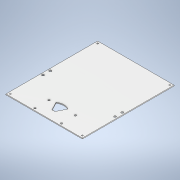
# Autodesk Inventor part: s_carbon_plate1
Saved by Autodesk Inventor 2022 (Build 260153000, 153)
## iProperties
Created: 2021-08-20
Part Number: s_carbon_plate1
Material: ABS プラスチック
Document SubType Name: Sheet Metal
Designer: yuta0
Density: 1.06 g/cm^3
Sheet Metal Rule: Default_mm
Appearance: 滑らか - 白
Author: yuta0
Autodesk Inventor part; units mm, degrees
ref_plane "YZ Plane" through (0, 0, 0) normal (1, 0, 0) x (0, 1, 0)
ref_plane "XZ Plane" through (0, 0, 0) normal (0, 1, 0) x (-1, 0, 0)
ref_plane "XY Plane" through (0, 0, 0) normal (0, 0, 1) x (1, 0, 0)
sketch "スケッチ1" plane through (0, 0, 0) normal (0, 1, 0) x (-1, 0, 0)
  line L0 (-87.5, 105) -> (87.5, 105)
  line L1 (87.5, 105) -> (87.5, -105)
  line L2 (87.5, -105) -> (-87.5, -105)
  line L3 (-87.5, -105) -> (-87.5, 105)
  line L4 (-87.5, 105) -> (87.5, -105) construction
  line L5 (87.5, 105) -> (-87.5, -105) construction
  point P0 (0, 0)
  dimension "d0" = 210
  dimension "d1" = 175
  measures "d0" distance of L0.end L1.end
  measures "d1" distance of L0.start L0.end
extrude "プレート1" add sketch "スケッチ1" along normal blind 2
sketch "スケッチ5" plane through (0, 2, 0) normal (0, 1, 0) x (1, 0, 0)
  line L0 (-26, -100) -> (34.6, -100)
  line L1 (34.6, -100) -> (34.6, -68)
  line L2 (34.6, -68) -> (-26, -68)
  line L3 (-26, -68) -> (-26, -100)
  line L4 (-26, -100) -> (34.6, -68) construction
  line L5 (34.6, -100) -> (-26, -68) construction
  line L6 (87.5, -105) -> (-87.5, -105) projected
  point P0 (0, 0)
  point P1 (0, -84)
  point P2 (4.3, -84)
  point P3 (4.3, -84)
  dimension "d31" = 60.6
  dimension "d32" = 26
  dimension "d33" = 32
  dimension "d34" = 21
  constraints: 12 end point, 3 midpoint, 2 parallel, 1 horizontal, 1 horizontal alignment, 1 perpendicular, 1 vertical alignment
  measures "d31" distance of L1.end L2.end
  measures "d32" distance from line of L3 point (0, -84)
  measures "d33" distance of L0.end L1.end
  measures "d34" distance from line of L6 point (0, -84)
hole "穴3" at (34.6, 2, 68) at (34.6, 2, 100) at (-26, 2, 68) at (-26, 2, 100) direction (0, -1, 0) diameter 4.3 end through all clearance for "Socket Head Cap Screw" size "M4" standard "Ansi Metric M Profile"
sketch "スケッチ6" plane through (0, 2, 0) normal (0, 1, 0) x (1, 0, 0)
  line L0 (-87.5, -251.5284) -> (85.7224, 84.4449)
  line L1 (85.7224, 84.4449) -> (87.5, 83.5284)
  line L2 (87.5, 83.5284) -> (-85.7224, -252.4449)
  line L3 (-85.7224, -252.4449) -> (-87.5, -251.5284)
  line L4 (-87.5, -251.5284) -> (87.5, 83.5284) construction
  line L5 (85.7224, 84.4449) -> (-85.7224, -252.4449) construction
  line L6 (87.5, -251.5284) -> (-85.7224, 84.4449)
  line L7 (-85.7224, 84.4449) -> (-87.5, 83.5284)
  line L8 (-87.5, 83.5284) -> (85.7224, -252.4449)
  line L9 (85.7224, -252.4449) -> (87.5, -251.5284)
  line L10 (87.5, -251.5284) -> (-87.5, 83.5284) construction
  line L11 (-85.7224, 84.4449) -> (85.7224, -252.4449) construction
  line L12 (-2.2636, -81.7918) -> (-0.486, -80.8753)
  circle A0 centre (0, -84) radius 22
  line L13 (2.2636, -81.7918) -> (0.486, -80.8753)
  circle A1 centre (0, -84) radius 3
  line L14 (-87.5, -105) -> (-87.5, 105) projected
  line L15 (87.5, 105) -> (87.5, -105) projected
  point P0 (0, 0)
  point P1 (0, -84)
  point P2 (-1.3748, -81.3335)
  point P3 (1.3748, -81.3335)
  point P4 (10.9601, -64.9245)
  point P5 (-10.9601, -64.9245)
  dimension "d54" = 2
  dimension "d55" = 2
  dimension "d57" = 44
  dimension "d59" = 3
  dimension "d60" = 3
  dimension "d65" = 186
  dimension "d66" = 186
  constraints: 28 end point, 6 point on line, 5 midpoint, 4 parallel, 4 perpendicular, 2 centre point, 2 coincident, 1 tangent
  measures "d54" distance between parallel lines of L6 L8
  measures "d55" distance between parallel lines of L0 L2
  measures "d57" diameter of A0
  measures "d59" distance from line of L12 A0.centre
  measures "d60" distance from line of L13 A0.centre
  measures "d65" distance between parallel lines of L7 L12
  measures "d66" distance between parallel lines of L1 L13
extrude "押し出し2" cut sketch "スケッチ6" against normal blind 10 contours A0 L6 L12 L8 | A0 L0 A1 L6 | L12 L6 A1 | A0 L2 L13 L0 | L0 L13 A1
sketch "スケッチ7" plane through (0, 2, 0) normal (0, 1, 0) x (1, 0, 0)
  line L0 (-82.5, -100) -> (82.5, -100)
  line L1 (82.5, -100) -> (82.5, 100)
  line L2 (82.5, 100) -> (-82.5, 100)
  line L3 (-82.5, 100) -> (-82.5, -100)
  line L4 (-82.5, -100) -> (82.5, 100) construction
  line L5 (82.5, -100) -> (-82.5, 100) construction
  line L6 (-87.5, -105) -> (-87.5, 105) projected
  line L7 (87.5, -105) -> (-87.5, -105) projected
  point P0 (0, 0)
  point P1 (-82.5, -25.14)
  point P2 (-82.5, -8.517)
  point P3 (82.5, -25.14)
  point P4 (82.5, -8.517)
  dimension "d45" = 5
  dimension "d46" = 5
  dimension "d67" = 74.86
  dimension "d68" = 16.623
  dimension "d69" = 74.86
  dimension "d70" = 16.623
  constraints: 12 end point, 4 point on line, 2 midpoint, 2 parallel, 1 horizontal, 1 perpendicular
  measures "d45" distance between parallel lines of L6 L3
  measures "d46" distance between parallel lines of L7 L0
  measures "d67" distance from line of L0 point (-82.5, -25.14)
  measures "d68" distance of point (-82.5, -8.517) point (-82.5, -25.14)
  measures "d69" distance from line of L0 point (82.5, -25.14)
  measures "d70" distance of point (82.5, -25.14) point (82.5, -8.517)
hole "穴4" at (-82.5, 2, -100) at (82.5, 2, -100) at (-82.5, 2, 100) at (82.5, 2, 100) direction (0, -1, 0) diameter 3.2 end through all clearance for "Socket Head Cap Screw" size "M3" standard "Ansi Metric M Profile"
sketch "スケッチ8" plane through (0, 2, 0) normal (0, 1, 0) x (1, 0, 0)
  line L0 (10.9601, -64.9245) -> (2.2636, -81.7918) projected
  line L1 (-1.3748, -81.3335) -> (-2.2636, -81.7918) projected
  arc A0 (1.3748, -81.3335) -> (-1.3748, -81.3335) centre (0, -84) ccw projected
  line L2 (2.2636, -81.7918) -> (1.3748, -81.3335) projected
  line L3 (-2.2636, -81.7918) -> (-10.9601, -64.9245) projected
  arc A1 (10.9601, -64.9245) -> (-10.9601, -64.9245) centre (0, -84) ccw projected
  line L4 (3.1247, -84.486) -> (13.5784, -64.2105)
  arc A2 (13.5784, -64.2105) -> (-13.5784, -64.2105) centre (0, -84) ccw
  line L5 (-13.5784, -64.2105) -> (-3.1247, -84.486)
  line L6 (-3.1247, -84.486) -> (-0.4583, -83.1112)
  arc A3 (0.4583, -83.1112) -> (-0.4583, -83.1112) centre (0, -84) ccw
  line L7 (0.4583, -83.1112) -> (3.1247, -84.486)
  point P0 (0, 0)
  dimension "d61" = 2
  constraints: 8 end point, 4 point on circle, 2 centre point, 5 other
  measures "d61" distance between parallel lines of L5 L3
extrude "押し出し3" cut sketch "スケッチ8" against normal blind 10 contours L0 L2 A0 L1 L3 A1 | L7 A3 L6 L5 A2 L4
fillet "コーナーR1" radius 1 4 edges at (-3.1247, 1, 84.486) (3.1247, 1, 84.486) (-13.5784, 1, 64.2105) (13.5784, 1, 64.2105)
hole "穴5" at (-82.5, 2, 25.14) at (-82.5, 2, 8.517) at (82.5, 2, 25.14) at (82.5, 2, 8.517) direction (0, -1, 0) diameter 5.2 end through all
equation "\"d40\" = Thickness"
equation "\"d60\" = d59"
equation "\"d66\" = d65"
equation "\"d69\" = d67"
equation "\"d70\" = d68"
equation "\"d76\" = Thickness"
equation "\"d2\" = Thickness"
equation "\"BendRadius\" = Thickness"
equation "\"BendReliefWidth\" = Thickness"
equation "\"BendReliefDepth\" = 0.5 * Thickness"
equation "\"CornerReliefSize\" = 4 * Thickness"
equation "\"MinimumRemnant\" = 2 * Thickness"
equation "\"TransitionRadius\" = BendRadius"
equation "\"JacobiRadiusSize\" = BendRadius"
equation "\"GapSize\" = Thickness"
equation "\"Thickness\" = 2"
